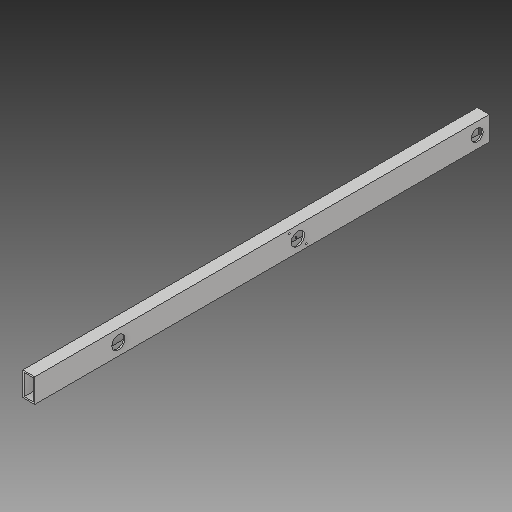
# Autodesk Inventor part: 34.48in Arm Bea
Saved by Autodesk Inventor 2018 (Build 220112000, 112)
## iProperties
Created: 2019-01-17
Part Number: 34.48in Arm Bea
Material: Generic
Document SubType Name: Modeling
Designer: Gabriel
Density: 1 g/cm^3
Appearance: Default
Author: Gabriel
Autodesk Inventor part; units mm, degrees
ref_plane "YZ Plane" through (0, 0, 0) normal (1, 0, 0) x (0, 1, 0)
ref_plane "XZ Plane" through (0, 0, 0) normal (0, 1, 0) x (-1, 0, 0)
ref_plane "XY Plane" through (0, 0, 0) normal (0, 0, 1) x (1, 0, 0)
sketch "Sketch1" plane through (0, 0, 0) normal (0, 0, 1) x (1, 0, 0)
  line L0 (-35.3228, 16.049) -> (-9.9228, 16.049)
  line L1 (-9.9228, 16.049) -> (-9.9228, -34.751)
  line L2 (-9.9228, -34.751) -> (-35.3228, -34.751)
  line L3 (-35.3228, -34.751) -> (-35.3228, 16.049)
  line L4 (-13.0978, 12.874) -> (-32.1478, 12.874)
  line L5 (-32.1478, 12.874) -> (-32.1478, -31.576)
  line L6 (-32.1478, -31.576) -> (-13.0978, -31.576)
  line L7 (-13.0978, -31.576) -> (-13.0978, 12.874)
  point P0 (0, 0)
  dimension "d0" = 25.4
  dimension "d1" = 50.8
  dimension "d2" = 3.175
  constraints: 16 end point, 4 parallel, 2 perpendicular, 1 horizontal, 3 other
  measures "d0" distance of L1.end L2.end
  measures "d1" distance of L0.end L1.end
  measures "d2" distance between parallel lines of L0 L4
extrude "Extrusion1" add sketch "Sketch1" along normal blind 965.2
sketch "Sketch2" plane through (-35.3228, -34.751, 0) normal (-1, 0, 0) x (0, 0, 1)
  line L0 (0, 0) -> (0, 50.8) construction
  line L1 (0, 25.4) -> (25.4, 25.4) construction
  circle A0 centre (25.4, 25.4) radius 12.7
  point P0 (0, 34.751)
  dimension "d5" = 25.4
  dimension "d9" = 25.4
  constraints: 2 end point, 1 centre point, 1 coincident, 1 horizontal, 1 midpoint
  measures "d5" distance of L1.start L1.end
  measures "d9" diameter of A0
extrude "Extrusion2" cut sketch "Sketch2" against normal blind 254
sketch "Sketch3" plane through (-35.3228, -34.751, 0) normal (-1, 0, 0) x (0, 0, 1)
  line L0 (965.2, 50.8) -> (965.2, 0) construction
  line L1 (965.2, 25.4) -> (787.4, 25.4) construction
  circle A0 centre (787.4, 25.4) radius 14.2875
  point P0 (0, 34.751)
  dimension "d10" = 177.8
  dimension "d11" = 28.575
  constraints: 2 end point, 1 centre point, 1 coincident, 1 horizontal, 1 midpoint
  measures "d10" distance of L1.start L1.end
  measures "d11" diameter of A0
extrude "Extrusion3" cut sketch "Sketch3" against normal blind 25.4
sketch "Sketch4" plane through (-35.3228, -34.751, 0) normal (-1, 0, 0) x (0, 0, 1)
  line L0 (965.2, 50.8) -> (965.2, 0) construction
  line L1 (965.2, 25.4) -> (406.4, 25.4) construction
  circle A0 centre (406.4, 25.4) radius 14.2875
  point P0 (0, 34.751)
  dimension "d14" = 558.8
  dimension "d15" = 28.575
  constraints: 2 end point, 1 centre point, 1 coincident, 1 horizontal, 1 midpoint
  measures "d14" distance of L1.start L1.end
  measures "d15" diameter of A0
extrude "Extrusion4" cut sketch "Sketch4" against normal blind 25.4
sketch "Sketch5" plane through (-35.3228, -34.751, 0) normal (-1, 0, 0) x (0, 0, 1)
  circle A0 centre (406.4, 25.4) radius 14.2875 construction
  line L0 (406.4, 25.4) -> (388.4395, 7.4395) construction
  line L1 (406.4, 25.4) -> (431.8, 25.4) construction
  line L2 (406.4, 25.4) -> (424.3605, 43.3605) construction
  circle A1 centre (388.4395, 7.4395) radius 2.032
  circle A2 centre (424.3605, 43.3605) radius 2.032
  point P0 (0, 34.751)
  dimension "d18" = 25.4
  dimension "d19" = 135
  dimension "d20" = 25.4
  dimension "d21" = 4.064
  dimension "d22" = 4.064
  constraints: 6 end point, 2 centre point, 2 coincident, 1 equal length, 1 horizontal
  measures "d18" distance of L0.start L0.end
  measures "d19" angle of L0 L1
  measures "d20" distance of L0.start L2.end
  measures "d21" diameter of A1
  measures "d22" diameter of A2
extrude "Extrusion5" cut sketch "Sketch5" against normal blind 25.4
body "Solid1"
